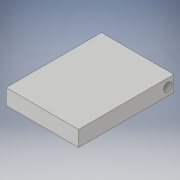
# Autodesk Inventor part: closing
Saved by Autodesk Inventor 2019 (Build 230136000, 136)
## iProperties
Created: 2020-02-28
Part Number: closing
Material: Generic
Document SubType Name: Modeling
Designer: LENOVO
Density: 1 g/cm^3
Appearance: Default
Author: LENOVO
Autodesk Inventor part; units mm, degrees
ref_plane "YZ Plane" through (0, 0, 0) normal (1, 0, 0) x (0, 1, 0)
ref_plane "XZ Plane" through (0, 0, 0) normal (0, 1, 0) x (-1, 0, 0)
ref_plane "XY Plane" through (0, 0, 0) normal (0, 0, 1) x (1, 0, 0)
sketch "Sketch1" plane through (0, 0, 0) normal (0, 0, 1) x (1, 0, 0)
  line L0 (0, 0) -> (20, 0)
  line L1 (20, 0) -> (20, 15)
  line L2 (20, 15) -> (0, 15)
  line L3 (0, 15) -> (0, 0)
  dimension "d0" = 20
  dimension "d1" = 15
  constraints: 8 end point, 2 parallel, 1 horizontal, 1 perpendicular
  measures "d0" distance of L2.end L1.end
  measures "d1" distance of L1.end L0.end
extrude "Extrusion1" add sketch "Sketch1" along normal blind 12
sketch "Sketch2" plane through (20, 0, 0) normal (1, 0, 0) x (0, 0, -1)
  circle A0 centre (-6, 7.5) radius 4
  point P0 (0, 0)
  dimension "d4" = 8
  constraints: 1 centre point
  measures "d4" diameter of A0
extrude "Extrusion2" cut sketch "Sketch2" against normal blind 10
sketch "Sketch3" plane through (0, 0, 12) normal (0, 0, 1) x (1, 0, 0)
  line L0 (4.6713, 10.3664) -> (9.2786, 10.3664)
  line L1 (9.2786, 10.3664) -> (9.2786, 7.6788)
  line L2 (9.2786, 7.6788) -> (4.6713, 7.6788)
  line L3 (4.6713, 7.6788) -> (4.6713, 10.3664)
  point P0 (0, 0)
  constraints: 8 end point, 2 parallel, 1 horizontal, 1 perpendicular
extrude "Extrusion3" add sketch "Sketch3" along normal blind 10
sketch "Sketch4" plane through (0, 0, 12) normal (0, 0, 1) x (1, 0, 0)
  line L0 (20, 0) -> (20, 15) projected
  line L1 (0, 15) -> (0, 0) projected
  line L2 (20, 15) -> (0, 15)
  line L3 (0, 15) -> (0, 0)
  line L4 (0, 0) -> (20, 0)
  line L5 (20, 0) -> (20, 15)
  constraints: 8 end point, 2 parallel, 1 horizontal, 1 perpendicular
extrude "Extrusion4" add sketch "Sketch4" along normal blind 50
sketch "Sketch5" plane through (0, 0, 0) normal (-1, 0, 0) x (0, 0, 1)
  line L0 (0, 15) -> (62, 15) projected
  line L1 (0, 0) -> (62, 0)
  line L2 (62, 0) -> (62, 15)
  line L3 (62, 15) -> (0, 15)
  line L4 (0, 15) -> (0, 0)
  constraints: 8 end point, 2 parallel, 1 horizontal, 1 perpendicular
extrude "Extrusion5" add sketch "Sketch5" along normal blind 50
sketch "Sketch6" plane through (0, 0, 62) normal (0, 0, 1) x (1, 0, 0)
  line L0 (20, 0) -> (20, 15) projected
  line L1 (20, 15) -> (-50, 15) projected
  line L2 (20, 0) -> (-50, 0)
  line L3 (-50, 0) -> (-50, 15)
  line L4 (-50, 15) -> (20, 15)
  line L5 (20, 15) -> (20, 0)
  point P0 (0, 0)
  constraints: 8 end point, 2 parallel, 1 horizontal, 1 perpendicular
extrude "Extrusion6" add sketch "Sketch6" along normal blind 30
body "Solid1"
